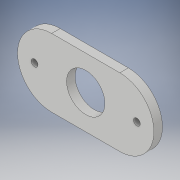
# Autodesk Inventor part: Bearing Plate
Saved by Autodesk Inventor 2019 (Build 230136000, 136)
## iProperties
Created: 2018-11-11
Part Number: Bearing Plate
Material: Generic
Document SubType Name: Modeling
Designer: maste
Density: 1 g/cm^3
Appearance: Default
Author: maste
Autodesk Inventor part; units mm, degrees
ref_plane "YZ Plane" through (0, 0, 0) normal (1, 0, 0) x (0, 1, 0)
ref_plane "XZ Plane" through (0, 0, 0) normal (0, 1, 0) x (-1, 0, 0)
ref_plane "XY Plane" through (0, 0, 0) normal (0, 0, 1) x (1, 0, 0)
sketch "Sketch1" plane through (0, 0, 0) normal (0, 0, 1) x (1, 0, 0)
  circle A0 centre (0, 0) radius 14.2875
  line L0 (0, 0) -> (38.1, 0)
  line L1 (0, 0) -> (-38.1, 0)
  circle A1 centre (-38.1, 0) radius 2.54
  circle A2 centre (38.1, 0) radius 2.54
  line L2 (38.1, 0) -> (50.8, 0)
  line L3 (50.8, 0) -> (50.8, 25.4)
  line L4 (-38.1, 0) -> (-50.8, 0)
  line L5 (50.8, 25.4) -> (-50.8, 25.4)
  line L6 (-50.8, 25.4) -> (-50.8, 0)
  line L7 (-50.8, 0) -> (-50.8, -25.4)
  line L8 (-50.8, -25.4) -> (50.8, -25.4)
  line L9 (50.8, -25.4) -> (50.8, 0)
  dimension "d0" = 28.575
  dimension "d1" = 38.1
  dimension "d2" = 38.1
  dimension "d3" = 5.08
  dimension "d4" = 5.08
  dimension "d6" = 12.7
  dimension "d7" = 25.4
  dimension "d8" = 12.7
  dimension "d9" = 25.4
  constraints: 20 end point, 5 horizontal, 3 centre point, 3 coincident, 3 perpendicular, 1 point on line, 1 vertical
  measures "d0" diameter of A0
  measures "d1" distance of L0.start L0.end
  measures "d2" distance of L0.start L1.end
  measures "d3" diameter of A1
  measures "d4" diameter of A2
  measures "d6" distance of L2.start L2.end
  measures "d7" distance of L2.end L3.end
  measures "d8" distance of L4.start L4.end
  measures "d9" distance of L4.end L7.end
extrude "Extrusion1" add sketch "Sketch1" along normal blind 6.35 contours L0 A2 L2 L9 L8 L7 L4 A1 L1 A0 | A0 L1 A1 L4 L6 L5 L3 L2 A2 L0
fillet "Fillet1" radius 25.4 4 edges at (50.8, 25.4, 3.175) (-50.8, 25.4, 3.175) (-50.8, -25.4, 3.175) (50.8, -25.4, 3.175)
body "Solid1"
